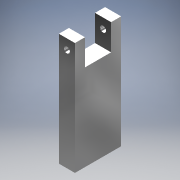
# Autodesk Inventor part: Gripper_Outer_Support_2
Saved by Autodesk Inventor 2021.3 (Build 253353000, 353)
## iProperties
Created: 2021-04-16
Part Number: Gripper_Outer_Support_2
Material: Aluminum 6061
Document SubType Name: Modeling
Designer: domin
Density: 2.7 g/cm^3
Appearance: Aluminum - Flat
Mass: 10.723 g
Surface Area: 23.6641 cm^2
Volume: 3.9715 cm^3
Author: domin
Autodesk Inventor part; units mm, degrees
ref_plane "YZ Plane" through (0, 0, 0) normal (1, 0, 0) x (0, 1, 0)
ref_plane "XZ Plane" through (0, 0, 0) normal (0, 1, 0) x (-1, 0, 0)
ref_plane "XY Plane" through (0, 0, 0) normal (0, 0, 1) x (1, 0, 0)
sketch "Sketch1" plane through (0, 0, 0) normal (1, 0, 0) x (0, 1, 0)
  line L0 (0, 11.5) -> (56, 11.5)
  line L1 (56, 11.5) -> (56, -11.5)
  line L2 (56, -11.5) -> (0, -11.5)
  line L3 (0, -11.5) -> (0, 11.5)
  point P0 (0, 0)
  dimension "d0" = 0
  dimension "d1" = 23
  dimension "d2" = 56
  dimension "d3" = 11.5
  constraints: 8 end point, 2 parallel, 1 horizontal, 1 perpendicular
  measures "d0" distance from line of point (0, 0) L3
  measures "d1" distance between parallel lines of L2 L0
  measures "d2" distance between parallel lines of L3 L1
  measures "d3" distance from line of point (0, 0) L0
extrude "Extrusion1" add sketch "Sketch1" along normal mid plane 8
sketch "Sketch2" plane through (4, 0, 0) normal (1, 0, 0) x (0, 0, -1)
  line L0 (11.5, 56) -> (-11.5, 56) projected
  line L1 (-6.5, 56) -> (6.5, 56)
  line L2 (6.5, 56) -> (6.5, 43)
  line L3 (6.5, 43) -> (-6.5, 43)
  line L4 (-6.5, 43) -> (-6.5, 56)
  point P0 (0, 0)
  dimension "d6" = 13
  dimension "d7" = 13
  dimension "d8" = 6.5
  constraints: 8 end point, 2 parallel, 1 horizontal, 1 perpendicular, 1 point on line
  measures "d6" distance of L2.end L3.end
  measures "d7" distance between parallel lines of L0 L3
  measures "d8" distance from line of point (0, 0) L4
extrude "Extrusion2" cut sketch "Sketch2" against normal through all
sketch "Sketch4" plane through (-4, 0, 11.5) normal (0, 0, 1) x (1, 0, 0)
  circle A0 centre (4, 51) radius 1.5
  line L0 (0, 56) -> (8, 56) projected
  line L1 (0, 0) -> (8, 0) projected
  point P0 (4, 0)
  point P1 (4, 0)
  dimension "d12" = 3
  dimension "d13" = 5
  constraints: 1 centre point, 1 midpoint, 1 vertical alignment
  measures "d12" diameter of A0
  measures "d13" distance from line of A0.centre L0
hole "Hole1" at (0, 51, 11.5) direction (0, 0, -1) diameter 3 end through all
sketch "Sketch5" plane through (-4, 0, -11.5) normal (0, -1, 0) x (1, 0, 0)
  circle A0 centre (4, 16.5) radius 1.5
  circle A1 centre (4, 6.5) radius 1.5
  point P0 (4, 11.5)
  dimension "d21" = 3
  dimension "d23" = 10
  dimension "d24" = 5
  constraints: 2 centre point, 2 vertical alignment, 1 equal radius
  measures "d21" diameter of A0
  measures "d23" distance of A1.centre A0.centre
  measures "d24" distance of A0.centre point (4, 11.5)
hole "Hole2" at (0, 0, 5) at (0, 0, -5) direction (0, 1, 0) diameter 2.459 depth 13 tip angle 118 thread size "M3x0.5" class "6H" standard "ISO Metric profile"
equation "\"d3\" = 0.5 * d1"
equation "\"d8\" = 0.5 * d6"
equation "\"d24\" = 0.5 * d23"
body "Solid1"
